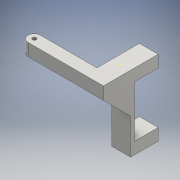
# Autodesk Inventor part: TurretServoSupport_A
Saved by Autodesk Inventor 2016 (Build 200138000, 138)
## iProperties
Created: 2016-04-17
Part Number: TurretServoSupport_A
Material: PC/ABS Plastic
Document SubType Name: Modeling
Designer: amenoni
Density: 0.357273 g/cm^3
Appearance: Smooth - White
Author: amenoni
Autodesk Inventor part; units mm, degrees
ref_plane "YZ Plane" through (0, 0, 0) normal (1, 0, 0) x (0, 1, 0)
ref_plane "XZ Plane" through (0, 0, 0) normal (0, 1, 0) x (-1, 0, 0)
ref_plane "XY Plane" through (0, 0, 0) normal (0, 0, 1) x (1, 0, 0)
sketch "Sketch1" plane through (0, 0, 0) normal (0, 1, 0) x (-1, 0, 0)
  line L0 (-7.5, -30) -> (7.5, -30)
  line L1 (7.5, -30) -> (7.5, 30)
  line L2 (7.5, 30) -> (-7.5, 30)
  line L3 (-7.5, 30) -> (-7.5, -30)
  line L4 (-7.5, -30) -> (7.5, 30) construction
  line L5 (7.5, -30) -> (-7.5, 30) construction
  point P0 (0, 0)
  dimension "d0" = 15
  dimension "d1" = 60
  constraints: 12 end point, 2 midpoint, 2 parallel, 1 horizontal, 1 perpendicular
  measures "d0" distance of L2.end L1.end
  measures "d1" distance of L1.end L0.end
extrude "Extrusion1" add sketch "Sketch1" along normal blind 3
sketch "Sketch2" plane through (0, 3, 0) normal (0, 1, 0) x (1, 0, 0)
  line L0 (-7.5, 30) -> (-7.5, -30) projected
  line L1 (7.5, 20.5) -> (-7.5, 20.5)
  line L2 (-7.5, 20.5) -> (-7.5, -20.5)
  line L3 (-7.5, -20.5) -> (7.5, -20.5)
  line L4 (7.5, -20.5) -> (7.5, 20.5)
  line L5 (7.5, 20.5) -> (-7.5, -20.5) construction
  line L6 (-7.5, 20.5) -> (7.5, -20.5) construction
  line L7 (7.5, -20.5) -> (-7.5, -20.5)
  line L8 (-7.5, -20.5) -> (-7.5, -30)
  line L9 (-7.5, -30) -> (7.5, -30)
  line L10 (7.5, -30) -> (7.5, -20.5)
  line L11 (7.5, 30) -> (-7.5, 30) projected
  line L12 (7.5, 20.5) -> (-7.5, 20.5)
  line L13 (-7.5, 20.5) -> (-7.5, 30)
  line L14 (-7.5, 30) -> (7.5, 30)
  line L15 (7.5, 30) -> (7.5, 20.5)
  point P0 (0, 0)
  dimension "d4" = 41
  constraints: 28 end point, 6 parallel, 3 horizontal, 3 perpendicular, 2 midpoint, 1 point on line
  measures "d4" distance of L2.end L1.end
extrude "Extrusion2" add sketch "Sketch2" along normal blind 19 contours L11 L15 L1 L0 | L3 L10 L9 L0
sketch "Sketch3" plane through (-7.5, 0, -30) normal (-1, 0, 0) x (0, 0, 1)
  line L0 (60, 0) -> (0, 0) projected
  line L1 (60, 0) -> (50, 0)
  line L2 (50, 0) -> (50, -21.64)
  line L3 (50, -21.64) -> (60, -21.64)
  line L4 (60, -21.64) -> (60, 0)
  point P0 (30, 0)
  dimension "d7" = 10
  dimension "d8" = 21.64
  constraints: 8 end point, 2 parallel, 1 horizontal, 1 perpendicular
  measures "d7" distance of L3.end L2.end
  measures "d8" distance of L2.end L1.end
extrude "Extrusion3" add sketch "Sketch3" against normal blind 15
sketch "Sketch5" plane through (-7.5, 0, -30) normal (-1, 0, 0) x (0, 0, 1)
  line L0 (0, 0) -> (50, 0) projected
  line L1 (28.3595, 0) -> (50, -21.6405)
  line L2 (50, -21.64) -> (50, 0) projected
  line L3 (28.3595, 0) -> (58.9638, 0) construction
  line L4 (50, -21.6405) -> (50, 0)
  line L5 (50, 0) -> (28.3595, 0)
  point P0 (30, 0)
  dimension "d15" = 45
  constraints: 8 end point, 2 collinear, 2 point on line, 1 equal length, 1 horizontal
  measures "d15" angle of L1 L3
extrude "Extrusion5" add sketch "Sketch5" against normal blind 15
sketch "Sketch6" plane through (-7.5, 0, -30) normal (-1, 0, 0) x (0, 0, 1)
  line L0 (60, -21.64) -> (60, 22) projected
  line L1 (60, -21.64) -> (50.1294, -21.64)
  line L2 (50.1294, -21.64) -> (50.1294, -11.769)
  line L3 (50.1294, -11.769) -> (60, -11.769)
  line L4 (60, -11.769) -> (60, -21.64)
  point P0 (30, 0)
  dimension "d18" = 9.871
  constraints: 8 end point, 2 parallel, 1 horizontal, 1 perpendicular
  measures "d18" distance of L1.end L2.end
extrude "Extrusion6" add sketch "Sketch6" along normal blind 50
sketch "Sketch7" plane through (-7.5, 22, 30) normal (0, 0, 1) x (1, 0, 0)
  point P0 (7.5, -22)
fillet "Fillet1" radius 5 2 edges at (-57.5, -21.64, 25.0647) (-57.5, -11.769, 25.0647)
sketch "Sketch8" plane through (-7.5, -21.64, 20.1294) normal (0, 0, -1) x (-1, 0, 0)
  arc A0 (45, 0) -> (50, 5) centre (45, 5) ccw projected
  point P0 (-7.5, 21.64)
  constraints: 1 coincident
hole "Hole1" at (-52.5, -16.64, 20.1294) direction (0, 0, 1) diameter 3 end through all
body "Solid1"
